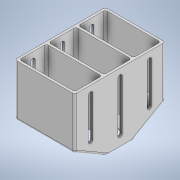
# Autodesk Inventor part: magazine-tower
Saved by Autodesk Inventor 2021 (Build 250183000, 183)
## iProperties
Created: 2024-03-15
Part Number: magazine-tower
Material: Generic
Document SubType Name: Modeling
Designer: 22hamfri
Density: 1 g/cm^3
Appearance: Default
Author: 22hamfri
Autodesk Inventor part; units mm, degrees
ref_plane "YZ Plane" through (0, 0, 0) normal (1, 0, 0) x (0, 1, 0)
ref_plane "XZ Plane" through (0, 0, 0) normal (0, 1, 0) x (-1, 0, 0)
ref_plane "XY Plane" through (0, 0, 0) normal (0, 0, 1) x (1, 0, 0)
sketch "Sketch1" plane through (0, 0, 0) normal (0, 1, 0) x (-1, 0, 0)
  line L0 (-24.5, 12) -> (24.5, 12)
  line L1 (24.5, 12) -> (24.5, -12)
  line L2 (24.5, -12) -> (-24.5, -12)
  line L3 (-24.5, -12) -> (-24.5, 12)
  line L4 (-24.5, 12) -> (24.5, -12) construction
  line L5 (24.5, 12) -> (-24.5, -12) construction
  line L6 (-26.5, 14) -> (26.5, 14)
  line L7 (26.5, 14) -> (26.5, -14)
  line L8 (26.5, -14) -> (-26.5, -14)
  line L9 (-26.5, -14) -> (-26.5, 14)
  line L10 (-26.5, 14) -> (26.5, -14) construction
  line L11 (26.5, 14) -> (-26.5, -14) construction
  point P0 (0, 0)
  dimension "d0" = 24
  dimension "d1" = 49
  dimension "d2" = 2
  dimension "d3" = 2
  constraints: 24 end point, 4 midpoint, 4 parallel, 2 horizontal, 2 perpendicular
  measures "d0" distance between parallel lines of L2 L0
  measures "d1" distance between parallel lines of L3 L1
  measures "d2" distance between parallel lines of L1 L7
  measures "d3" distance between parallel lines of L8 L2
extrude "Extrusion1" add sketch "Sketch1" along normal blind 60
sketch "Sketch2" plane through (26.5, 0, 14) normal (1, 0, 0) x (0, 0, -1)
  line L0 (0, 0) -> (28, 0) projected
  line L1 (28, 0) -> (28, 60) projected
  line L2 (0, 60) -> (28, 60) projected
  line L3 (0, 0) -> (0, 60) projected
  line L4 (26, 0) -> (2, 0) projected
  line L5 (2, 0) -> (2, 60) projected
  line L6 (26, 60) -> (2, 60) projected
  line L7 (26, 0) -> (26, 60) projected
  line L8 (2, 0) -> (2, 60) projected
  line L9 (2, 1.1547) -> (26, 1.1547)
  line L10 (26, 0) -> (26, 60) projected
  line L11 (2, 1.1547) -> (0, 1.1547)
  line L12 (0, 0) -> (0, 60) projected
  line L13 (26, 1.1547) -> (28, 1.1547)
  line L14 (28, 0) -> (28, 60) projected
  line L15 (28, 16.1658) -> (52, 16.1658)
  line L16 (52, 16.1658) -> (54, 16.1658)
  line L17 (52, 16.1658) -> (26, 1.1547)
  line L18 (52, 16.1658) -> (52, 60)
  line L19 (52, 60) -> (28, 60)
  line L20 (52, 60) -> (54, 60)
  line L21 (54, 60) -> (54, 16.1658)
  line L22 (54, 16.1658) -> (54, 15.0111)
  line L23 (54, 15.0111) -> (28, 0)
  line L24 (28, 0) -> (0, 0)
  point P0 (14, 0)
  point P1 (28, 2.3094)
  dimension "d6" = 2
  dimension "d8" = 30
  dimension "d15" = 0
  constraints: 26 end point, 8 point on line, 7 perpendicular, 3 parallel, 2 vertical, 1 horizontal
  measures "d6" distance between parallel lines of L23 L17
  measures "d8" angle of L9 L17
  measures "d15" distance between parallel lines of L24 L4
extrude "Extrusion2" add sketch "Sketch2" against normal up to surface (53 mm away) contours L1 L17 L16 L22 L23 | L16 L18 L20 L21
extrude "Extrusion3" add sketch "Sketch2" against normal up to surface (2 mm away) contours L1 L15 L17 | L19 L18 L15 L1
sketch "Sketch3" plane through (-26.5, 0, -14) normal (-1, 0, 0) x (0, 0, 1)
  line L0 (0, 0) -> (28, 0) projected
  line L1 (28, 0) -> (28, 60) projected
  line L2 (0, 60) -> (28, 60) projected
  line L3 (0, 2.3094) -> (0, 60) projected
  line L4 (-24, 16.1658) -> (0, 2.3094) projected
  line L5 (-24, 60) -> (-24, 16.1658) projected
  line L6 (-26, 60) -> (-24, 60) projected
  line L7 (-26, 15.0111) -> (-26, 60) projected
  line L8 (0, 0) -> (-26, 15.0111) projected
  line L9 (0, 60) -> (28, 60) projected
  line L10 (-26, 60) -> (-24, 60) projected
  line L11 (0, 60) -> (-24, 60)
  point P0 (14, 0)
  constraints: 2 end point, 1 horizontal
extrude "Extrusion4" add sketch "Sketch3" against normal up to surface (2 mm away) contours L3 L4 L5 L11
sketch "Sketch4" plane through (24.5, 2.3094, -14) normal (-1, 0, 0) x (0, 0, 1)
  line L0 (-24, 57.6906) -> (0, 57.6906) projected
  line L1 (-24, 13.8564) -> (-24, 57.6906) projected
  line L2 (0, 0) -> (-24, 13.8564) projected
  line L3 (0, 57.6906) -> (0, 0) projected
  line L4 (2, -2.3094) -> (26, -2.3094) projected
  line L5 (26, -2.3094) -> (26, 57.6906) projected
  line L6 (2, 57.6906) -> (26, 57.6906) projected
  line L7 (2, -2.3094) -> (2, 57.6906) projected
  line L8 (0, 0) -> (2, -1.1547)
  line L9 (2, -2.3094) -> (2, 57.6906) projected
  line L10 (0, 57.6906) -> (0, 0) projected
  line L11 (0, 11) -> (2, 9.8453)
  point P0 (14, -2.3094)
  dimension "d20" = 11
  constraints: 4 end point, 3 point on line, 1 collinear, 1 parallel
  measures "d20" distance of L11.start L2.start
extrude "Extrusion5" cut sketch "Sketch4" along normal up to surface (49 mm away) contours L11 L7 L8 L3
mirror "Mirror1" about plane through (0, 0, 0) normal (0, 0, 1) of "Extrusion2", "Extrusion3", "Extrusion4", "Extrusion5"
fillet "Fillet1" radius 2 12 edges at (24.5, 36.6547, -14) (24.5, 38.0829, -38) (-24.5, 38.0829, -38) (-24.5, 36.6547, -14) (-24.5, 36.0774, 12) (-24.5, 36.0774, -12) (24.5, 36.0774, -12) (24.5, 36.0774, 12) (24.5, 38.0829, 38) (24.5, 36.6547, 14) (-24.5, 36.6547, 14) (-24.5, 38.0829, 38)
fillet "Fillet2" radius 2 4 edges at (-26.5, 37.5056, -40) (26.5, 37.5056, -40) (26.5, 37.5056, 40) (-26.5, 37.5056, 40)
fillet "Fillet3" radius 2 10 edges at (-25.9142, 14.6729, -39.4142) (0, 15.0111, -40) (25.9142, 14.6729, -39.4142) (26.5, 6.9282, -26) (-26.5, 6.9282, -26) (-25.9142, 14.6729, 39.4142) (0, 15.0111, 40) (25.9142, 14.6729, 39.4142) (26.5, 6.9282, 26) (-26.5, 6.9282, 26)
sketch "Sketch5" plane through (26.5, 60, 38) normal (1, 0, 0) x (0, 0, -1)
  line L0 (0, 0) -> (0, -43.8342) projected
  line L1 (0, -43.8342) -> (0, 0) projected
  line L2 (24, -46.6906) -> (24, 0) projected
  line L3 (24, 0) -> (24, -46.6906) projected
  line L4 (50, 0) -> (50, -47.8453) projected
  line L5 (50, -47.8453) -> (50, 0) projected
  line L6 (76, -43.8342) -> (76, 0) projected
  line L7 (76, 0) -> (76, -43.8342) projected
  line L8 (26, -47.8453) -> (26, 0) projected
  line L9 (26, 0) -> (26, -47.8453) projected
  line L10 (52, 0) -> (52, -46.6906) projected
  line L11 (52, -46.6906) -> (52, 0) projected
  line L12 (0, -43.8342) -> (0, 0) projected
  line L13 (0, -5) -> (76, -5)
  line L14 (76, 0) -> (76, -43.8342) projected
  line L15 (2, -44.9889) -> (0, -43.8342) projected
  line L16 (0, -43.8342) -> (2, -44.9889) projected
  line L17 (2, -44.9889) -> (26, -58.8453) projected
  line L18 (2, -44.9889) -> (26, -58.8453) projected
  line L19 (76, -43.8342) -> (74, -44.9889) projected
  line L20 (74, -44.9889) -> (50, -58.8453) projected
  line L21 (50, -58.8453) -> (74, -44.9889) projected
  line L22 (74, -44.9889) -> (76, -43.8342) projected
  line L23 (24, -46.6906) -> (24, -57.6906)
  line L24 (28, -60) -> (0, -43.8342) projected
  line L25 (26, -47.8453) -> (26, -58.8453)
  line L26 (50, -47.8453) -> (50, -58.8453)
  line L27 (52, -46.6906) -> (52, -57.6906)
  line L28 (76, -43.8342) -> (48, -60) projected
  line L29 (0, 0) -> (76, 0) projected
  line L30 (28, -60) -> (0, -43.8342) projected
  line L31 (28, -60) -> (48, -60) projected
  line L32 (76, -43.8342) -> (48, -60) projected
  line L33 (76, 0) -> (76, -43.8342) projected
  line L34 (0, 0) -> (76, 0) projected
  line L35 (0, -43.8342) -> (0, 0) projected
  line L36 (26, -53.0718) -> (50, -53.0718)
  line L37 (50, -53.0718) -> (76, -38.0607)
  line L38 (76, -43.8342) -> (76, 0) projected
  line L39 (26, -53.0718) -> (0, -38.0607)
  line L40 (38, -53.0718) -> (38, -5)
  line L41 (64, -5) -> (64, -44.9889)
  line L42 (52, -46.6906) -> (52, 0) projected
  line L43 (52, -5) -> (64, -5)
  line L44 (64, -5) -> (76, -5)
  line L45 (66, -5) -> (66, -43.8342)
  line L46 (62, -5) -> (62, -46.1436)
  line L47 (62, -5) -> (64, -5)
  line L48 (64, -5) -> (66, -5)
  line L49 (36, -5) -> (36, -53.0718)
  line L50 (40, -53.0718) -> (40, -5)
  line L51 (36, -5) -> (38, -5)
  line L52 (38, -5) -> (40, -5)
  line L53 (12, -5) -> (12, -44.9889)
  line L54 (10, -5) -> (10, -43.8342)
  line L55 (14, -5) -> (14, -46.1436)
  line L56 (14, -5) -> (12, -5)
  line L57 (12, -5) -> (10, -5)
  point P0 (38, -60)
  point P1 (12, -5)
  point P2 (10, -5)
  point P3 (14, -5)
  dimension "d26" = 5
  dimension "d27" = 5
  dimension "d28" = 4
  dimension "d29" = 4
  constraints: 50 end point, 31 point on line, 10 symmetric about line, 7 perpendicular, 7 vertical, 6 collinear, 2 midpoint, 10 other
  measures "d26" distance of the line from the sketch origin of L13
  measures "d27" distance between parallel lines of L37 L32
  measures "d28" distance between parallel lines of L50 L49
  measures "d29" distance between parallel lines of L45 L46
extrude "Extrusion6" cut sketch "Sketch5" against normal up to surface (2 mm away) contours L13 L53 L39 L54 | L13 L55 L39 L53 | L13 L40 L36 L49 | L13 L50 L36 L40 | L13 L41 L37 L46 | L13 L45 L37 L41
fillet "Fillet4" radius 2 12 edges at (25.5, 16.1658, 28) (25.5, 13.8564, 24) (25.5, 55, 28) (25.5, 55, 24) (25.5, 55, -2) (25.5, 55, -28) (25.5, 55, -24) (25.5, 55, 2) (25.5, 16.1658, -28) (25.5, 13.8564, -24) (25.5, 6.9282, 2) (25.5, 6.9282, -2)
mirror "Mirror2" about plane through (0, 0, 0) normal (1, 0, 0) of "Extrusion6", "Fillet4"
equation "\"d29\" = d28"
body "Solid1"
